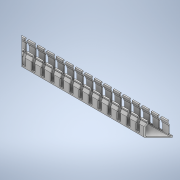
# Autodesk Inventor part: Cuerpo 30x30 317mm
Saved by Autodesk Inventor 2021 (Build 250183000, 183)
## iProperties
Created: 2021-04-16
Part Number: Cuerpo 30x30 317mm
Material: Generic
Document SubType Name: Modeling
Designer: Nelson
Density: 1 g/cm^3
Appearance: Default
Author: Nelson
Autodesk Inventor part; units mm, degrees
ref_plane "YZ Plane" through (0, 0, 0) normal (1, 0, 0) x (0, 1, 0)
ref_plane "XZ Plane" through (0, 0, 0) normal (0, 1, 0) x (-1, 0, 0)
ref_plane "XY Plane" through (0, 0, 0) normal (0, 0, 1) x (1, 0, 0)
sketch "Boceto principal" plane through (0, 0, 0) normal (1, 0, 0) x (0, 1, 0)
  line L0 (0, -1) -> (0, -29)
  line L1 (1, -30) -> (20, -30)
  line L2 (20, -30) -> (26, -27)
  line L3 (26, -27) -> (28, -27)
  line L4 (28, -27) -> (28, -28)
  line L5 (28, -28) -> (30, -28)
  line L6 (30, -28) -> (30, -25)
  line L7 (30, -25) -> (26, -25)
  line L8 (26, -25) -> (20, -28)
  line L9 (20, -28) -> (3, -28)
  line L10 (2, -27) -> (2, -3)
  line L11 (3, -2) -> (20, -2)
  line L12 (20, -2) -> (26, -5)
  line L13 (26, -5) -> (30, -5)
  line L14 (30, -5) -> (30, -2)
  line L15 (30, -2) -> (28, -2)
  line L16 (28, -2) -> (28, -3)
  line L17 (28, -3) -> (26, -3)
  line L18 (26, -3) -> (20, 0)
  line L19 (20, 0) -> (1, 0)
  arc A0 (1, 0) -> (0, -1) centre (1, -1) ccw
  arc A1 (0, -29) -> (1, -30) centre (1, -29) ccw
  arc A2 (2, -27) -> (3, -28) centre (3, -27) ccw
  arc A3 (3, -2) -> (2, -3) centre (3, -3) ccw
  constraints: 40 end point, 8 point on circle, 4 centre point
extrude "Extrusion1" add sketch "Boceto principal" along normal blind 317
sketch "Boceto agujeros" plane through (0, 0, 0) normal (0, 0, 1) x (1, 0, 0)
  line L0 (11, 4) -> (17, 4)
  line L1 (18, 5) -> (18, 18)
  line L2 (17, 19) -> (11, 19)
  line L3 (10, 18) -> (10, 5)
  line L4 (17, 19) -> (17, 30)
  line L5 (17, 30) -> (11, 30)
  line L6 (11, 19) -> (11, 30)
  arc A0 (10, 5) -> (11, 4) centre (11, 5) ccw
  arc A1 (17, 4) -> (18, 5) centre (17, 5) ccw
  arc A2 (18, 18) -> (17, 19) centre (17, 18) ccw
  arc A3 (11, 19) -> (10, 18) centre (11, 18) ccw
  constraints: 14 end point, 8 point on circle, 4 centre point
extrude "Extrusion2" cut sketch "Boceto agujeros" against normal blind 125
pattern_linear "Rectangular Pattern1" count 20 spacing 20 along (1, 0, 0) of "Extrusion2"
sketch "Boceto esquinas" plane through (0, 0, 0) normal (0, 1, 0) x (-1, 0, 0)
  line L0 (0, 0) -> (-30, 0)
  line L1 (-30, 0) -> (0, -30)
  line L2 (0, -30) -> (0, 0)
  line L3 (-287, 0) -> (-317, 0)
  line L4 (-317, 0) -> (-317, -30)
  line L5 (-317, -30) -> (-287, 0)
  constraints: 12 end point
extrude "Extrusion3" cut sketch "Boceto esquinas" along normal blind 30
body "Solid1"
